Autodesk Inventor part; units mm, degrees
(part 2 of 2)
sketch "스케치10" plane through (0, 0, 19) normal (0, 0, 1) x (1, 0, 0)
  line L0 (4.2, 30.6) -> (-4.2, 30.6) projected
  line L1 (-4.5, 30.6) -> (-4.5, 33.6515) projected
  line L2 (4.5, 33.6515) -> (4.5, 30.6) projected
  line L3 (2.4, 34.3) -> (4.9, 34.3) projected
  arc A0 (4.6757, 34.0757) -> (4.5, 33.6515) centre (5.1, 33.6515) ccw projected
  line L4 (4.9, 34.3) -> (4.6757, 34.0757) projected
  arc A1 (2, 34.7) -> (2.4, 34.3) centre (2.4, 34.7) ccw projected
  line L5 (2, 35.3) -> (2, 34.7) projected
  circle A2 centre (0, 0) radius 37 projected
  arc A3 (-7.2608, 33.6199) -> (-7.2809, 33.1611) centre (-6.717, 33.3663) ccw projected
  line L6 (-7.2809, 33.1611) -> (-6.2372, 30.2937) projected
  line L7 (-6.2372, 30.2937) -> (-4.5, 30.6) projected
  line L8 (-4.5, 30.6) -> (-4.5, 33.6515) projected
  arc A4 (-4.5, 33.6515) -> (-4.6757, 34.0757) centre (-5.1, 33.6515) ccw projected
  line L9 (-4.6757, 34.0757) -> (-4.9, 34.3) projected
  line L10 (-4.9, 34.3) -> (-2.4, 34.3) projected
  arc A5 (-2.4, 34.3) -> (-2, 34.7) centre (-2.4, 34.7) ccw projected
  line L11 (-2, 34.7) -> (-2, 35.3) projected
  line L12 (-2, 35.3) -> (2, 35.3) projected
  line L13 (2, 35.3) -> (2, 34.7) projected
  arc A6 (2, 34.7) -> (2.4, 34.3) centre (2.4, 34.7) ccw projected
  line L14 (2.4, 34.3) -> (4.9, 34.3) projected
  line L15 (4.9, 34.3) -> (4.6757, 34.0757) projected
  arc A7 (4.6757, 34.0757) -> (4.5, 33.6515) centre (5.1, 33.6515) ccw projected
  line L16 (4.5, 33.6515) -> (4.5, 30.6) projected
  line L17 (4.5, 30.6) -> (6.2372, 30.2937) projected
  line L18 (6.2372, 30.2937) -> (7.2809, 33.1611) projected
  arc A8 (7.2809, 33.1611) -> (7.2608, 33.6199) centre (6.717, 33.3663) ccw projected
  line L19 (7.2608, 33.6199) -> (7.1268, 33.9074) projected
  line L20 (7.1268, 33.9074) -> (9.476, 33.0523) projected
  arc A9 (9.476, 33.0523) -> (9.9887, 33.2914) centre (9.6128, 33.4282) ccw projected
  line L21 (9.9887, 33.2914) -> (10.1939, 33.8552) projected
  line L22 (10.1939, 33.8552) -> (13.9527, 32.4871) projected
  line L23 (13.9527, 32.4871) -> (13.7475, 31.9233) projected
  arc A10 (13.7475, 31.9233) -> (13.9866, 31.4106) centre (14.1234, 31.7865) ccw projected
  line L24 (13.9866, 31.4106) -> (16.3358, 30.5556) projected
  line L25 (16.3358, 30.5556) -> (16.0483, 30.4215) projected
  arc A11 (16.0483, 30.4215) -> (15.7381, 30.0829) centre (16.3019, 29.8777) ccw projected
  line L26 (15.7381, 30.0829) -> (14.6944, 27.2155) projected
  line L27 (14.6944, 27.2155) -> (16.2221, 26.3335) projected
  line L28 (16.2221, 26.3335) -> (18.1835, 28.6711) projected
  arc A12 (18.1835, 28.6711) -> (18.3216, 29.109) centre (17.7239, 29.0567) ccw projected
  line L29 (18.3216, 29.109) -> (18.294, 29.425) projected
  line L30 (18.294, 29.425) -> (20.2091, 27.818) projected
  arc A13 (20.2091, 27.818) -> (20.7726, 27.8673) centre (20.4662, 28.1244) ccw projected
  line L31 (20.7726, 27.8673) -> (21.1583, 28.3269) projected
  line L32 (21.1583, 28.3269) -> (24.2225, 25.7558) projected
  line L33 (24.2225, 25.7558) -> (23.8368, 25.2962) projected
  arc A14 (23.8368, 25.2962) -> (23.8861, 24.7326) centre (24.1432, 25.0391) ccw projected
  line L34 (23.8861, 24.7326) -> (25.8012, 23.1257) projected
  line L35 (25.8012, 23.1257) -> (25.4853, 23.098) projected
  arc A15 (25.4853, 23.098) -> (25.0779, 22.886) centre (25.5376, 22.5003) ccw projected
  line L36 (25.0779, 22.886) -> (23.1165, 20.5484) projected
  line L37 (23.1165, 20.5484) -> (24.2504, 19.1971) projected
  line L38 (24.2504, 19.1971) -> (26.893, 20.7229) projected
  arc A16 (26.893, 20.7229) -> (27.1726, 21.0872) centre (26.593, 21.2425) ccw projected
  line L39 (27.1726, 21.0872) -> (27.2547, 21.3935) projected
  line L40 (27.2547, 21.3935) -> (28.5047, 19.2285) projected
  arc A17 (28.5047, 19.2285) -> (29.0511, 19.0821) centre (28.8511, 19.4285) ccw projected
  line L41 (29.0511, 19.0821) -> (29.5707, 19.3821) projected
  line L42 (29.5707, 19.3821) -> (31.5707, 15.9179) projected
  line L43 (31.5707, 15.9179) -> (31.0511, 15.6179) projected
  arc A18 (31.0511, 15.6179) -> (30.9047, 15.0715) centre (31.2511, 15.2715) ccw projected
  line L44 (30.9047, 15.0715) -> (32.1547, 12.9065) projected
  line L45 (32.1547, 12.9065) -> (31.8483, 12.9886) projected
  arc A19 (31.8483, 12.9886) -> (31.393, 12.9286) centre (31.693, 12.409) ccw projected
  line L46 (31.393, 12.9286) -> (28.7504, 11.4029) projected
  line L47 (28.7504, 11.4029) -> (29.3537, 9.7453) projected
  line L48 (29.3537, 9.7453) -> (32.3588, 10.2752) projected
  arc A20 (32.3588, 10.2752) -> (32.7461, 10.5219) centre (32.2546, 10.866) ccw projected
  line L49 (32.7461, 10.5219) -> (32.928, 10.7817) projected
  line L50 (32.928, 10.7817) -> (33.3622, 8.3197) projected
  arc A21 (33.3622, 8.3197) -> (33.8255, 7.9952) centre (33.7561, 8.3891) ccw projected
  line L51 (33.8255, 7.9952) -> (34.4164, 8.0994) projected
  line L52 (34.4164, 8.0994) -> (35.111, 4.1602) projected
  line L53 (35.111, 4.1602) -> (34.5201, 4.056) projected
  arc A22 (34.5201, 4.056) -> (34.1957, 3.5926) centre (34.5896, 3.6621) ccw projected
  line L54 (34.1957, 3.5926) -> (34.6298, 1.1306) projected
  line L55 (34.6298, 1.1306) -> (34.37, 1.3125) projected
  arc A23 (34.37, 1.3125) -> (33.9216, 1.4119) centre (34.0258, 0.821) ccw projected
  line L56 (33.9216, 1.4119) -> (30.9165, 0.882) projected
  line L57 (30.9165, 0.882) -> (30.9165, -0.882) projected
  line L58 (30.9165, -0.882) -> (33.9216, -1.4119) projected
  arc A24 (33.9216, -1.4119) -> (34.37, -1.3125) centre (34.0258, -0.821) ccw projected
  line L59 (34.37, -1.3125) -> (34.6298, -1.1306) projected
  line L60 (34.6298, -1.1306) -> (34.1957, -3.5926) projected
  arc A25 (34.1957, -3.5926) -> (34.5201, -4.056) centre (34.5896, -3.6621) ccw projected
  line L61 (34.5201, -4.056) -> (35.111, -4.1602) projected
  line L62 (35.111, -4.1602) -> (34.4164, -8.0994) projected
  line L63 (34.4164, -8.0994) -> (33.8255, -7.9952) projected
  arc A26 (33.8255, -7.9952) -> (33.3622, -8.3197) centre (33.7561, -8.3891) ccw projected
  line L64 (33.3622, -8.3197) -> (32.928, -10.7817) projected
  line L65 (32.928, -10.7817) -> (32.7461, -10.5219) projected
  arc A27 (32.7461, -10.5219) -> (32.3588, -10.2752) centre (32.2546, -10.866) ccw projected
  line L66 (32.3588, -10.2752) -> (29.3537, -9.7453) projected
  line L67 (29.3537, -9.7453) -> (28.7504, -11.4029) projected
  line L68 (28.7504, -11.4029) -> (31.393, -12.9286) projected
  arc A28 (31.393, -12.9286) -> (31.8483, -12.9886) centre (31.693, -12.409) ccw projected
  line L69 (31.8483, -12.9886) -> (32.1547, -12.9065) projected
  line L70 (32.1547, -12.9065) -> (30.9047, -15.0715) projected
  arc A29 (30.9047, -15.0715) -> (31.0511, -15.6179) centre (31.2511, -15.2715) ccw projected
  line L71 (31.0511, -15.6179) -> (31.5707, -15.9179) projected
  line L72 (31.5707, -15.9179) -> (29.5707, -19.3821) projected
  line L73 (29.5707, -19.3821) -> (29.0511, -19.0821) projected
  arc A30 (29.0511, -19.0821) -> (28.5047, -19.2285) centre (28.8511, -19.4285) ccw projected
  line L74 (28.5047, -19.2285) -> (27.2547, -21.3935) projected
  line L75 (27.2547, -21.3935) -> (27.1726, -21.0872) projected
  arc A31 (27.1726, -21.0872) -> (26.893, -20.7229) centre (26.593, -21.2425) ccw projected
  line L76 (26.893, -20.7229) -> (24.2504, -19.1971) projected
  line L77 (24.2504, -19.1971) -> (23.1165, -20.5484) projected
  line L78 (23.1165, -20.5484) -> (25.0779, -22.886) projected
  arc A32 (25.0779, -22.886) -> (25.4853, -23.098) centre (25.5376, -22.5003) ccw projected
  line L79 (25.4853, -23.098) -> (25.8012, -23.1257) projected
  line L80 (25.8012, -23.1257) -> (23.8861, -24.7326) projected
  arc A33 (23.8861, -24.7326) -> (23.8368, -25.2962) centre (24.1432, -25.0391) ccw projected
  line L81 (23.8368, -25.2962) -> (24.2225, -25.7558) projected
  line L82 (24.2225, -25.7558) -> (21.1583, -28.3269) projected
  line L83 (21.1583, -28.3269) -> (20.7726, -27.8673) projected
  arc A34 (20.7726, -27.8673) -> (20.2091, -27.818) centre (20.4662, -28.1244) ccw projected
  line L84 (20.2091, -27.818) -> (18.294, -29.425) projected
  line L85 (18.294, -29.425) -> (18.3216, -29.109) projected
  arc A35 (18.3216, -29.109) -> (18.1835, -28.6711) centre (17.7239, -29.0567) ccw projected
  line L86 (18.1835, -28.6711) -> (16.2221, -26.3335) projected
  line L87 (16.2221, -26.3335) -> (14.6944, -27.2155) projected
  line L88 (14.6944, -27.2155) -> (15.7381, -30.0829) projected
  arc A36 (15.7381, -30.0829) -> (16.0483, -30.4215) centre (16.3019, -29.8777) ccw projected
  line L89 (16.0483, -30.4215) -> (16.3358, -30.5556) projected
  line L90 (16.3358, -30.5556) -> (13.9866, -31.4106) projected
  arc A37 (13.9866, -31.4106) -> (13.7475, -31.9233) centre (14.1234, -31.7865) ccw projected
  line L91 (13.7475, -31.9233) -> (13.9527, -32.4871) projected
  line L92 (13.9527, -32.4871) -> (10.1939, -33.8552) projected
  line L93 (10.1939, -33.8552) -> (9.9887, -33.2914) projected
  arc A38 (9.9887, -33.2914) -> (9.476, -33.0523) centre (9.6128, -33.4282) ccw projected
  line L94 (9.476, -33.0523) -> (7.1268, -33.9074) projected
  line L95 (7.1268, -33.9074) -> (7.2608, -33.6199) projected
  arc A39 (7.2608, -33.6199) -> (7.2809, -33.1611) centre (6.717, -33.3663) ccw projected
  line L96 (7.2809, -33.1611) -> (6.2372, -30.2937) projected
  line L97 (6.2372, -30.2937) -> (4.5, -30.6) projected
  line L98 (4.5, -30.6) -> (4.5, -33.6515) projected
  arc A40 (4.5, -33.6515) -> (4.6757, -34.0757) centre (5.1, -33.6515) ccw projected
  line L99 (4.6757, -34.0757) -> (4.9, -34.3) projected
  line L100 (4.9, -34.3) -> (2.4, -34.3) projected
  arc A41 (2.4, -34.3) -> (2, -34.7) centre (2.4, -34.7) ccw projected
  line L101 (2, -34.7) -> (2, -35.3) projected
  line L102 (2, -35.3) -> (-2, -35.3) projected
  line L103 (-2, -35.3) -> (-2, -34.7) projected
  arc A42 (-2, -34.7) -> (-2.4, -34.3) centre (-2.4, -34.7) ccw projected
  line L104 (-2.4, -34.3) -> (-4.9, -34.3) projected
  line L105 (-4.9, -34.3) -> (-4.6757, -34.0757) projected
  arc A43 (-4.6757, -34.0757) -> (-4.5, -33.6515) centre (-5.1, -33.6515) ccw projected
  line L106 (-4.5, -33.6515) -> (-4.5, -30.6) projected
  line L107 (-4.5, -30.6) -> (-6.2372, -30.2937) projected
  line L108 (-6.2372, -30.2937) -> (-7.2809, -33.1611) projected
  arc A44 (-7.2809, -33.1611) -> (-7.2608, -33.6199) centre (-6.717, -33.3663) ccw projected
  line L109 (-7.2608, -33.6199) -> (-7.1268, -33.9074) projected
  line L110 (-7.1268, -33.9074) -> (-9.476, -33.0523) projected
  arc A45 (-9.476, -33.0523) -> (-9.9887, -33.2914) centre (-9.6128, -33.4282) ccw projected
  line L111 (-9.9887, -33.2914) -> (-10.1939, -33.8552) projected
  line L112 (-10.1939, -33.8552) -> (-13.9527, -32.4871) projected
  line L113 (-13.9527, -32.4871) -> (-13.7475, -31.9233) projected
  arc A46 (-13.7475, -31.9233) -> (-13.9866, -31.4106) centre (-14.1234, -31.7865) ccw projected
  line L114 (-13.9866, -31.4106) -> (-16.3358, -30.5556) projected
  line L115 (-16.3358, -30.5556) -> (-16.0483, -30.4215) projected
  arc A47 (-16.0483, -30.4215) -> (-15.7381, -30.0829) centre (-16.3019, -29.8777) ccw projected
  line L116 (-15.7381, -30.0829) -> (-14.6944, -27.2155) projected
  line L117 (-14.6944, -27.2155) -> (-16.2221, -26.3335) projected
  line L118 (-16.2221, -26.3335) -> (-18.1835, -28.6711) projected
  arc A48 (-18.1835, -28.6711) -> (-18.3216, -29.109) centre (-17.7239, -29.0567) ccw projected
  line L119 (-18.3216, -29.109) -> (-18.294, -29.425) projected
  line L120 (-18.294, -29.425) -> (-20.2091, -27.818) projected
  arc A49 (-20.2091, -27.818) -> (-20.7726, -27.8673) centre (-20.4662, -28.1244) ccw projected
  line L121 (-20.7726, -27.8673) -> (-21.1583, -28.3269) projected
  line L122 (-21.1583, -28.3269) -> (-24.2225, -25.7558) projected
  line L123 (-24.2225, -25.7558) -> (-23.8368, -25.2962) projected
  arc A50 (-23.8368, -25.2962) -> (-23.8861, -24.7326) centre (-24.1432, -25.0391) ccw projected
  line L124 (-23.8861, -24.7326) -> (-25.8012, -23.1257) projected
  line L125 (-25.8012, -23.1257) -> (-25.4853, -23.098) projected
  arc A51 (-25.4853, -23.098) -> (-25.0779, -22.886) centre (-25.5376, -22.5003) ccw projected
  line L126 (-25.0779, -22.886) -> (-23.1165, -20.5484) projected
  line L127 (-23.1165, -20.5484) -> (-24.2504, -19.1971) projected
  line L128 (-24.2504, -19.1971) -> (-26.893, -20.7229) projected
  arc A52 (-26.893, -20.7229) -> (-27.1726, -21.0872) centre (-26.593, -21.2425) ccw projected
  line L129 (-27.1726, -21.0872) -> (-27.2547, -21.3935) projected
  line L130 (-27.2547, -21.3935) -> (-28.5047, -19.2285) projected
  arc A53 (-28.5047, -19.2285) -> (-29.0511, -19.0821) centre (-28.8511, -19.4285) ccw projected
  line L131 (-29.0511, -19.0821) -> (-29.5707, -19.3821) projected
  line L132 (-29.5707, -19.3821) -> (-31.5707, -15.9179) projected
  line L133 (-31.5707, -15.9179) -> (-31.0511, -15.6179) projected
  arc A54 (-31.0511, -15.6179) -> (-30.9047, -15.0715) centre (-31.2511, -15.2715) ccw projected
  line L134 (-30.9047, -15.0715) -> (-32.1547, -12.9065) projected
  line L135 (-32.1547, -12.9065) -> (-31.8483, -12.9886) projected
  arc A55 (-31.8483, -12.9886) -> (-31.393, -12.9286) centre (-31.693, -12.409) ccw projected
  line L136 (-31.393, -12.9286) -> (-28.7504, -11.4029) projected
  line L137 (-28.7504, -11.4029) -> (-29.3537, -9.7453) projected
  line L138 (-29.3537, -9.7453) -> (-32.3588, -10.2752) projected
  arc A56 (-32.3588, -10.2752) -> (-32.7461, -10.5219) centre (-32.2546, -10.866) ccw projected
  line L139 (-32.7461, -10.5219) -> (-32.928, -10.7817) projected
  line L140 (-32.928, -10.7817) -> (-33.3622, -8.3197) projected
  arc A57 (-33.3622, -8.3197) -> (-33.8255, -7.9952) centre (-33.7561, -8.3891) ccw projected
  line L141 (-33.8255, -7.9952) -> (-34.4164, -8.0994) projected
  line L142 (-34.4164, -8.0994) -> (-35.111, -4.1602) projected
  line L143 (-35.111, -4.1602) -> (-34.5201, -4.056) projected
  arc A58 (-34.5201, -4.056) -> (-34.1957, -3.5926) centre (-34.5896, -3.6621) ccw projected
  line L144 (-34.1957, -3.5926) -> (-34.6298, -1.1306) projected
  line L145 (-34.6298, -1.1306) -> (-34.37, -1.3125) projected
  arc A59 (-34.37, -1.3125) -> (-33.9216, -1.4119) centre (-34.0258, -0.821) ccw projected
  line L146 (-33.9216, -1.4119) -> (-30.9165, -0.882) projected
  line L147 (-30.9165, -0.882) -> (-30.9165, 0.882) projected
  line L148 (-30.9165, 0.882) -> (-33.9216, 1.4119) projected
  arc A60 (-33.9216, 1.4119) -> (-34.37, 1.3125) centre (-34.0258, 0.821) ccw projected
  line L149 (-34.37, 1.3125) -> (-34.6298, 1.1306) projected
  line L150 (-34.6298, 1.1306) -> (-34.1957, 3.5926) projected
  arc A61 (-34.1957, 3.5926) -> (-34.5201, 4.056) centre (-34.5896, 3.6621) ccw projected
  line L151 (-34.5201, 4.056) -> (-35.111, 4.1602) projected
  line L152 (-35.111, 4.1602) -> (-34.4164, 8.0994) projected
  line L153 (-34.4164, 8.0994) -> (-33.8255, 7.9952) projected
  arc A62 (-33.8255, 7.9952) -> (-33.3622, 8.3197) centre (-33.7561, 8.3891) ccw projected
  line L154 (-33.3622, 8.3197) -> (-32.928, 10.7817) projected
  line L155 (-32.928, 10.7817) -> (-32.7461, 10.5219) projected
  arc A63 (-32.7461, 10.5219) -> (-32.3588, 10.2752) centre (-32.2546, 10.866) ccw projected
  line L156 (-32.3588, 10.2752) -> (-29.3537, 9.7453) projected
  line L157 (-29.3537, 9.7453) -> (-28.7504, 11.4029) projected
  line L158 (-28.7504, 11.4029) -> (-31.393, 12.9286) projected
  arc A64 (-31.393, 12.9286) -> (-31.8483, 12.9886) centre (-31.693, 12.409) ccw projected
  line L159 (-31.8483, 12.9886) -> (-32.1547, 12.9065) projected
  line L160 (-32.1547, 12.9065) -> (-30.9047, 15.0715) projected
  arc A65 (-30.9047, 15.0715) -> (-31.0511, 15.6179) centre (-31.2511, 15.2715) ccw projected
  line L161 (-31.0511, 15.6179) -> (-31.5707, 15.9179) projected
  line L162 (-31.5707, 15.9179) -> (-29.5707, 19.3821) projected
  line L163 (-29.5707, 19.3821) -> (-29.0511, 19.0821) projected
  arc A66 (-29.0511, 19.0821) -> (-28.5047, 19.2285) centre (-28.8511, 19.4285) ccw projected
  line L164 (-28.5047, 19.2285) -> (-27.2547, 21.3935) projected
  line L165 (-27.2547, 21.3935) -> (-27.1726, 21.0872) projected
  arc A67 (-27.1726, 21.0872) -> (-26.893, 20.7229) centre (-26.593, 21.2425) ccw projected
  line L166 (-26.893, 20.7229) -> (-24.2504, 19.1971) projected
  line L167 (-24.2504, 19.1971) -> (-23.1165, 20.5484) projected
  line L168 (-23.1165, 20.5484) -> (-25.0779, 22.886) projected
  arc A68 (-25.0779, 22.886) -> (-25.4853, 23.098) centre (-25.5376, 22.5003) ccw projected
  line L169 (-25.4853, 23.098) -> (-25.8012, 23.1257) projected
  line L170 (-25.8012, 23.1257) -> (-23.8861, 24.7326) projected
  arc A69 (-23.8861, 24.7326) -> (-23.8368, 25.2962) centre (-24.1432, 25.0391) ccw projected
  line L171 (-23.8368, 25.2962) -> (-24.2225, 25.7558) projected
  line L172 (-24.2225, 25.7558) -> (-21.1583, 28.3269) projected
  line L173 (-21.1583, 28.3269) -> (-20.7726, 27.8673) projected
  arc A70 (-20.7726, 27.8673) -> (-20.2091, 27.818) centre (-20.4662, 28.1244) ccw projected
  line L174 (-20.2091, 27.818) -> (-18.294, 29.425) projected
  line L175 (-18.294, 29.425) -> (-18.3216, 29.109) projected
  arc A71 (-18.3216, 29.109) -> (-18.1835, 28.6711) centre (-17.7239, 29.0567) ccw projected
  line L176 (-18.1835, 28.6711) -> (-16.2221, 26.3335) projected
  line L177 (-16.2221, 26.3335) -> (-14.6944, 27.2155) projected
  line L178 (-14.6944, 27.2155) -> (-15.7381, 30.0829) projected
  arc A72 (-15.7381, 30.0829) -> (-16.0483, 30.4215) centre (-16.3019, 29.8777) ccw projected
  line L179 (-16.0483, 30.4215) -> (-16.3358, 30.5556) projected
  line L180 (-16.3358, 30.5556) -> (-13.9866, 31.4106) projected
  arc A73 (-13.9866, 31.4106) -> (-13.7475, 31.9233) centre (-14.1234, 31.7865) ccw projected
  line L181 (-13.7475, 31.9233) -> (-13.9527, 32.4871) projected
  line L182 (-13.9527, 32.4871) -> (-10.1939, 33.8552) projected
  line L183 (-10.1939, 33.8552) -> (-9.9887, 33.2914) projected
  arc A74 (-9.9887, 33.2914) -> (-9.476, 33.0523) centre (-9.6128, 33.4282) ccw projected
  line L184 (-9.476, 33.0523) -> (-7.1268, 33.9074) projected
  line L185 (-7.1268, 33.9074) -> (-7.2608, 33.6199) projected
